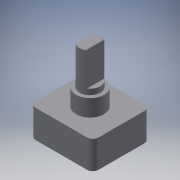
# Autodesk Inventor part: Потенциометр
Saved by Autodesk Inventor 2019.1 (Build 231200000, 200)
## iProperties
Created: 2018-07-27
Part Number: Потенциометр
Material: Типовые
Document SubType Name: Modeling
Designer: olege
Density: 1 g/cm^3
Appearance: По умолчанию
Author: olege
Autodesk Inventor part; units mm, degrees
ref_plane "YZ Plane" through (0, 0, 0) normal (1, 0, 0) x (0, 1, 0)
ref_plane "XZ Plane" through (0, 0, 0) normal (0, 1, 0) x (-1, 0, 0)
sketch "Эскиз1" plane through (0, 0, 0) normal (0, 0, 1) x (1, 0, 0)
  line L0 (-5.6, 5.1) -> (5.6, 5.1)
  line L1 (5.6, 5.1) -> (5.6, -5.1)
  line L2 (5.6, -5.1) -> (-5.6, -5.1)
  line L3 (-5.6, -5.1) -> (-5.6, 5.1)
  line L4 (-5.6, 5.1) -> (5.6, -5.1) construction
  line L5 (5.6, 5.1) -> (-5.6, -5.1) construction
  point P0 (0, 0)
  dimension "d0" = 11.2
  dimension "d1" = 10.2
  constraints: 12 end point, 2 midpoint, 2 parallel, 1 horizontal, 1 perpendicular
  measures "d0" distance of L1.end L2.end
  measures "d1" distance of L0.end L1.end
extrude "Выдавливание1" add sketch "Эскиз1" along normal blind 5
fillet "Сопряжение1" radius 1 4 edges at (-5.6, 5.1, 2.5) (5.6, 5.1, 2.5) (5.6, -5.1, 2.5) (-5.6, -5.1, 2.5)
sketch "Эскиз2" plane through (0, 0, 5) normal (0, 0, 1) x (1, 0, 0)
  circle A0 centre (0, 0) radius 2.5
  dimension "d5" = 5
  constraints: 1 centre point, 1 coincident
  measures "d5" diameter of A0
extrude "Выдавливание2" add sketch "Эскиз2" along normal blind 3
sketch "Эскиз3" plane through (0, 0, 8) normal (0, 0, 1) x (1, 0, 0)
  circle A0 centre (0, 0) radius 1.85
  dimension "d8" = 3.7
  constraints: 1 centre point, 1 coincident
  measures "d8" diameter of A0
extrude "Выдавливание3" add sketch "Эскиз3" along normal blind 7
sketch "Эскиз4" plane through (0, 0, 15) normal (0, 0, 1) x (1, 0, 0)
  line L0 (1, -5) -> (-1, -5)
  line L1 (-1, -5) -> (-1, 5)
  line L2 (-1, 5) -> (1, 5)
  line L3 (1, 5) -> (1, -5)
  line L4 (1, -5) -> (-1, 5) construction
  line L5 (-1, -5) -> (1, 5) construction
  line L6 (-1, 5) -> (-9.7743, 5)
  line L7 (-9.7743, 5) -> (-9.7743, -5)
  line L8 (-9.7743, -5) -> (-1, -5)
  line L9 (-1, -5) -> (-1, 5)
  line L10 (1, -5) -> (12.6944, -5)
  line L11 (12.6944, -5) -> (12.6944, 8.8009)
  line L12 (12.6944, 8.8009) -> (1, 8.8009)
  line L13 (1, 8.8009) -> (1, -5)
  point P0 (0, 0)
  dimension "d11" = 2
  dimension "d12" = 10
  constraints: 28 end point, 6 parallel, 3 horizontal, 3 perpendicular, 2 midpoint
  measures "d11" distance of L1.end L2.end
  measures "d12" distance of L0.end L1.end
extrude "Выдавливание4" cut sketch "Эскиз4" against normal blind 6 contours L3 L13 L12 L11 L10 | L8 L7 L6 L1
fillet "Сопряжение2" radius 0.2 4 edges at (0, -1.85, 15) (0, 1.85, 15) (1, 0, 15) (-1, 0, 15)
ref_plane "РабПлоскость1" through (0, 0, 8) normal (0, 0, 1) x (1, 0, 0)
